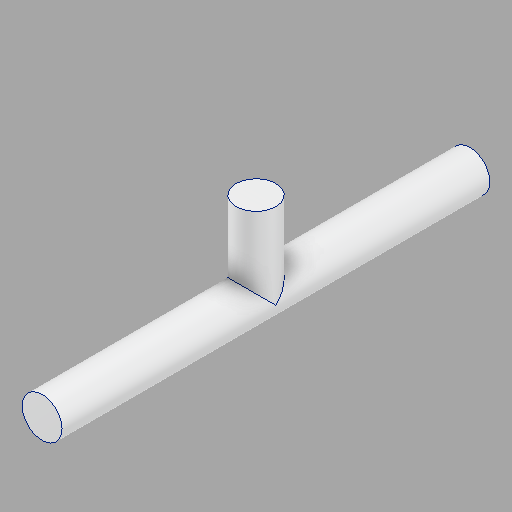
# Autodesk Inventor part: Ось_антенны
Saved by Autodesk Inventor 2025 (Build 290162000, 162)
## iProperties
Created: 2024-11-27
Part Number: Ось_антенны
Material: Алюминий 6061
Document SubType Name: Modeling
Designer: Artem Sannikov
Density: 2.7 g/cm^3
Appearance: Алюминий — плоский
Author: Artem Sannikov
Autodesk Inventor part; units mm, degrees
ref_plane "YZ Plane" through (0, 0, 0) normal (1, 0, 0) x (0, 1, 0)
ref_plane "XZ Plane" through (0, 0, 0) normal (0, 1, 0) x (-1, 0, 0)
ref_plane "XY Plane" through (0, 0, 0) normal (0, 0, 1) x (1, 0, 0)
sketch "Эскиз1" plane through (0, 0, 0) normal (0, 0, 1) x (1, 0, 0)
  circle A0 centre (0, 0) radius 3.5
  dimension "d0" = 7
  constraints: 1 centre point, 1 coincident
  measures "d0" diameter of A0
extrude "Выдавливание1" add sketch "Эскиз1" along normal blind 75
sketch "Эскиз2" plane through (0, 0, 0) normal (0, 1, 0) x (-1, 0, 0)
  line L0 (3.5, 75) -> (-3.5, 75) projected
  line L1 (0, 75) -> (0, 0) construction
  circle A0 centre (0, 37.5) radius 3.5
  constraints: 2 end point, 2 midpoint, 1 centre point, 1 vertical
extrude "Выдавливание2" add sketch "Эскиз2" along normal blind 15
